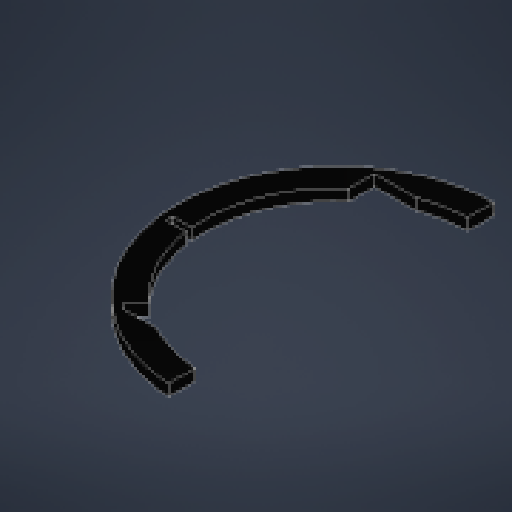
# Autodesk Inventor part: Front_aligner
Saved by Autodesk Inventor 2023 (Build 270158000, 158)
## iProperties
Created: 2023-05-07
Part Number: Front_aligner
Material: Generic
Document SubType Name: Modeling
Designer: szykr
Density: 1 g/cm^3
Appearance: Anodized - Black
Author: szykr
Autodesk Inventor part; units mm, degrees
ref_plane "YZ Plane" through (0, 0, 0) normal (1, 0, 0) x (0, 1, 0)
ref_plane "XZ Plane" through (0, 0, 0) normal (0, 1, 0) x (-1, 0, 0)
ref_plane "XY Plane" through (0, 0, 0) normal (0, 0, 1) x (1, 0, 0)
sketch "Sketch1" plane through (0, 0, 0) normal (0, 1, 0) x (-1, 0, 0)
  circle A0 centre (0, 0) radius 40 projected
  circle A1 centre (0, 0) radius 35 projected
  line L0 (2.3, 32.9859) -> (2.3, 40) projected
  line L1 (21.9637, 27.3435) -> (25.5064, 30.8949) projected
  line L2 (21.9637, 27.3435) -> (21.9123, 27.292)
  line L3 (26.5671, 29.8368) -> (23.0244, 26.2855) projected
  line L4 (26.5671, 29.8368) -> (26.6021, 29.8719)
  line L5 (25.4356, 30.9655) -> (21.8929, 27.4142)
  line L6 (21.8929, 27.4142) -> (21.8415, 27.3626)
  line L7 (21.8415, 27.3626) -> (21.8337, 27.3548)
  line L8 (23.0952, 26.2148) -> (26.6379, 29.7662)
  line L9 (26.6379, 29.7662) -> (26.6729, 29.8013)
  line L10 (26.6729, 29.8013) -> (26.6768, 29.8052)
  circle A2 centre (0, 0) radius 42
  line L11 (2.4, 32.9859) -> (2.4, 39.9955)
  line L12 (34.7391, 5.0137) -> (39.7719, 5.0137) projected
  line L13 (39.7719, 3.5174) -> (34.7391, 3.5174) projected
  line L14 (34.7391, 5.1137) -> (39.7645, 5.1137)
  line L15 (39.7719, 3.4174) -> (34.7391, 3.4174)
  line L16 (34.7391, 5.1137) -> (34.6244, 5.1137)
  line L17 (39.7719, 3.4174) -> (39.8538, 3.4174)
  line L18 (23, -32.7261) -> (23, -26.3818) projected
  line L19 (23.1, -32.7236) -> (23.1, -26.3856)
  line L20 (23.1, -26.3856) -> (23.1, -26.2943)
  line L21 (21.5, -32.7261) -> (21.5, -26.3818) projected
  line L22 (21.4, -32.723) -> (21.4, -26.3818)
  line L23 (21.4, -32.723) -> (21.4, -33.7941)
  line L24 (0.75, -35) -> (0.75, -40) projected
  line L25 (0.85, -35.0011) -> (0.85, -39.8733)
  line L26 (0.85, -35.0011) -> (0.85, -34.9897)
  line L27 (0.85, -39.8733) -> (0.85, -41.9914)
  line L28 (2.4, 39.9955) -> (2.4, 41.9314)
  line L29 (23, -32.7261) -> (21.5, -32.7261) projected
  line L30 (22.8571, -32.8261) -> (21.4, -32.8261)
  line L31 (23.1, -32.7236) -> (23.1, -32.8261)
  line L32 (22.8571, -32.8261) -> (23.1, -32.8261)
  line L33 (39.7719, 5.0137) -> (39.7719, 3.5174) projected
  line L34 (39.8719, 3.4174) -> (39.8719, 5.1137)
  line L35 (39.7645, 5.1137) -> (39.8719, 5.1137)
  line L36 (39.8719, 3.4174) -> (39.8538, 3.4174)
  point P0 (2.4, 34.9176)
  point P1 (25.3839, 30.9137)
  point P2 (23.1396, 26.2594)
  point P3 (39.6718, 5.1137)
  point P4 (34.8328, 3.4174)
  point P5 (23.1, -32.6556)
  point P6 (21.4, -27.6955)
  dimension "d0" = 0.1
  dimension "d1" = 0.1
  dimension "d2" = 2
  dimension "d3" = 0.1
  dimension "d4" = 0.1
  dimension "d5" = 0.1
  dimension "d6" = 0.1
  dimension "d7" = 0.1
  dimension "d8" = 0.1
  dimension "d13" = 0.1
  dimension "d16" = 0.1
  constraints: 54 end point, 12 collinear, 12 point on circle, 7 parallel, 3 horizontal, 3 point on line, 1 centre point, 2 other
  measures "d0" distance between parallel lines of L1 L5
  measures "d1" distance between parallel lines of L3 L8
  measures "d2" radial gap between concentric circles of A0 A2
  measures "d3" distance between parallel lines of L0 L11
  measures "d4" distance between parallel lines of L12 L14
  measures "d5" distance between parallel lines of L13 L15
  measures "d6" distance between parallel lines of L18 L19
  measures "d7" distance between parallel lines of L21 L22
  measures "d8" distance between parallel lines of L24 L25
  measures "d13" distance between parallel lines of L29 L30
  measures "d16" distance between parallel lines of L33 L34
extrude "Extrusion1" add sketch "Sketch1" along normal blind 3 contours A0 L19 L20 A1 L15 L17 | A0 L36 L34 L35 L14 L11 L28 A2 L27 L32 L31 L19 | L14 L16 A1 L8 L9 L10 A0 | A0 L27 L25 L26 A1 L22 L23 | L5 L6 L7 A1 L11 A0
sketch "Sketch2" plane through (0, 3, 0) normal (0, 1, 0) x (1, 0, 0)
  line L0 (-21.4, 33.7941) -> (-21.4, 27.6955) projected
  arc A0 (-0.85, 34.9897) -> (-21.4, 27.6955) centre (0, 0) ccw projected
  line L1 (-25.3839, -30.9137) -> (-16.4117, -30.9137)
  arc A1 (-21.8337, -27.3548) -> (-2.4, -34.9176) centre (0, 0) ccw projected
  line L2 (-21.8337, -27.3548) -> (-25.3839, -30.9137) projected
  line L3 (-23.1, 32.8261) -> (-12.1427, 32.8261)
  point P0 (-9.1082, 33.7941)
  point P1 (-21.4, 32.8261)
  constraints: 4 end point, 3 point on circle, 2 horizontal
extrude "Extrusion2" cut sketch "Sketch2" against normal through all
sketch "Sketch3" plane through (0, 3, 0) normal (0, 1, 0) x (1, 0, 0)
  line L0 (-21.4, 33.7941) -> (-21.4, 32.8261) projected
  line L1 (-22.8571, 32.8261) -> (-21.4, 32.8261)
  arc A0 (-21.4, 33.7941) -> (-22.8571, 32.8261) centre (0, 0) ccw projected
  constraints: 2 end point, 1 horizontal
extrude "Extrusion3" add sketch "Sketch3" against normal blind 3
equation "\"d0\" = slack"
equation "\"d1\" = slack"
equation "\"d3\" = slack"
equation "\"d4\" = slack"
equation "\"d5\" = slack"
equation "\"d6\" = slack"
equation "\"d7\" = slack"
equation "\"d8\" = slack"
equation "\"d13\" = slack"
equation "\"d16\" = slack"
equation "\"d9\" = thicc"
equation "\"d14\" = thicc"
equation "\"slack\" = 0.1"
equation "\"thicc\" = 3"
body "Solid1"
